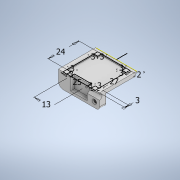
# Autodesk Inventor part: DisplayClipBase
Saved by Autodesk Inventor 2020.3 (Build 243373000, 373)
## iProperties
Created: 2020-07-13
Part Number: DisplayClipBase
Material: Generisch
Document SubType Name: Modeling
Designer: hpcwoess
Density: 1 g/cm^3
Appearance: Vorgabe
Author: hpcwoess
Autodesk Inventor part; units mm, degrees
ref_plane "YZ Plane" through (0, 0, 0) normal (1, 0, 0) x (0, 1, 0)
ref_plane "XZ Plane" through (0, 0, 0) normal (0, 1, 0) x (-1, 0, 0)
ref_plane "XY Plane" through (0, 0, 0) normal (0, 0, 1) x (1, 0, 0)
sketch "Skizze1" plane through (0, 0, 0) normal (0, 0, 1) x (1, 0, 0)
  line L0 (0, 0) -> (-11.6, 0)
  line L1 (-11.6, 0) -> (-11.6, 1.6)
  line L2 (-11.6, 1.6) -> (-9.6, 1.6)
  line L3 (-9.6, 1.6) -> (-9.6, 4.2)
  line L4 (-9.6, 4.2) -> (-16, 4.2)
  line L5 (-16, 4.2) -> (-16, 7)
  line L6 (-16, 7) -> (0, 7)
  line L7 (0, 7) -> (0, 0)
  dimension "d0" = 9.6
  dimension "d1" = 11.6
  dimension "d2" = 1.6
  dimension "d3" = 4.2
  dimension "d4" = 7
  dimension "d5" = 16
  constraints: 16 end point, 7 perpendicular, 1 horizontal
  measures "d0" distance between parallel lines of L7 L3
  measures "d1" distance of L0.start L0.end
  measures "d2" distance from line of L0.start L2
  measures "d3" distance between parallel lines of L4 L0
  measures "d4" distance between parallel lines of L0 L6
  measures "d5" distance between parallel lines of L7 L5
extrude "Extrusion1" add sketch "Skizze1" along normal blind 24
mirror "Spiegeln1" about plane through (0, 0, 0) normal (1, 0, 0) of "Extrusion1"
sketch "Skizze2" plane through (0, 0, 24) normal (0, 0, 1) x (1, 0, 0)
  line L0 (-16, 7) -> (-16, 4.2) projected
  line L1 (-16, 7) -> (16, 7)
  line L2 (16, 7) -> (16, -5)
  line L3 (16, -5) -> (-16, -5)
  line L4 (-16, -5) -> (-16, 7)
  line L5 (16, 7) -> (16, 4.2) projected
  point P0 (0, 0)
  dimension "d8" = 12
  constraints: 8 end point, 2 parallel, 1 collinear, 1 horizontal, 1 perpendicular
  measures "d8" distance between parallel lines of L3 L1
extrude "Extrusion2" add sketch "Skizze2" along normal blind 5
sketch "Skizze3" plane through (0, 0, 0) normal (1, 0, 0) x (0, 1, 0)
  line L0 (0, 0) -> (0, 24) projected
  line L1 (0.3, 3.5) -> (1.6, 3.5)
  line L2 (1.6, 3.5) -> (0, 11.5)
  line L3 (0, 11.5) -> (0, 4.0745)
  line L4 (1.6, 0) -> (0, 0) projected
  line L5 (0.3, 3.5) -> (0.3, 0)
  line L6 (0, 0) -> (0, 4.0745)
  line L7 (-5, 24) -> (4.2, 24) projected
  point P0 (0, 11.5)
  dimension "d12" = 8
  dimension "d13" = 1.7
  dimension "d14" = 0.3
  dimension "d20" = 20.5
  dimension "d65" = 1.3
  constraints: 10 end point, 2 perpendicular, 2 point on line, 1 horizontal, 1 vertical
  measures "d12" distance from line of L1 L2.end
  measures "d13" distance of L3.end L1.end
  measures "d14" distance between parallel lines of L0 L5
  measures "d20" distance between parallel lines of L1 L7
  measures "d65" distance of L1.start L1.end
extrude "Extrusion3" cut sketch "Skizze3" against normal mid plane 14
sketch "Skizze4" plane through (-16, 7, 0) normal (0, 1, 0) x (1, 0, 0)
  line L0 (3.5, -2) -> (28.5, -2)
  line L1 (28.5, -2) -> (28.5, -29)
  line L2 (28.5, -29) -> (3.5, -29)
  line L3 (3.5, -29) -> (3.5, -2)
  line L4 (16, 0) -> (16, 8.5337)
  line L5 (32, 0) -> (0, 0) projected
  line L6 (9.5, -26) -> (22.5, -26)
  line L7 (22.5, -26) -> (22.5, -29)
  line L8 (22.5, -29) -> (9.5, -29)
  line L9 (9.5, -29) -> (9.5, -26)
  line L10 (3.5, -29) -> (6.5, -29)
  line L11 (6.5, -29) -> (6.5, -26)
  line L12 (6.5, -26) -> (3.5, -26)
  line L13 (3.5, -26) -> (3.5, -29)
  line L14 (3.5, -2) -> (6.5, -2)
  line L15 (6.5, -2) -> (6.5, -5)
  line L16 (6.5, -5) -> (3.5, -5)
  line L17 (3.5, -5) -> (3.5, -2)
  line L18 (28.5, -29) -> (25.5, -29)
  line L19 (25.5, -29) -> (25.5, -26)
  line L20 (25.5, -26) -> (28.5, -26)
  line L21 (28.5, -26) -> (28.5, -29)
  line L22 (28.5, -2) -> (25.5, -2)
  line L23 (25.5, -2) -> (25.5, -5)
  line L24 (25.5, -5) -> (28.5, -5)
  line L25 (28.5, -5) -> (28.5, -2)
  point P0 (3.5, -26)
  dimension "d17" = 25
  dimension "d18" = 27
  dimension "d19" = 2
  dimension "d21" = 3
  dimension "d22" = 13
  dimension "d23" = 24
  dimension "d24" = 3
  dimension "d25" = 3
  dimension "d26" = 3
  dimension "d27" = 3
  dimension "d28" = 3
  dimension "d29" = 3
  dimension "d30" = 3
  dimension "d31" = 3
  constraints: 50 end point, 12 parallel, 6 horizontal, 6 perpendicular, 1 vertical, 2 other
  measures "d17" distance of L1.end L2.end
  measures "d18" distance of L0.end L1.end
  measures "d19" distance between parallel lines of L5 L0
  measures "d21" distance of L6.end L7.end
  measures "d22" distance of L7.end L8.end
  measures "d23" distance between parallel lines of L0 L6
  measures "d24" distance of L12.end L11.end
  measures "d25" distance of L11.end L10.end
  measures "d26" distance of L15.end L16.end
  measures "d27" distance of L14.end L15.end
  measures "d28" distance of L19.end L20.end
  measures "d29" distance of L18.end L19.end
  measures "d30" distance of L24.end L23.end
  measures "d31" distance of L23.end L22.end
extrude "Extrusion4" cut sketch "Skizze4" against normal blind 1 contours L0 L23 L24 L1 L20 L19 L2 L7 L6 L9 L11 L12 L3 L16 L15
extrude "Extrusion5" cut sketch "Skizze4" against normal blind 10 contours L9 L6 L7 L2
sketch "Skizze5" plane through (0, 0, 29) normal (0, 0, 1) x (1, 0, 0)
  circle A0 centre (12, -1) radius 1.75
  line L0 (-16, -5) -> (16, -5) projected
  line L1 (16, -5) -> (16, 7) projected
  point P0 (0, 0)
  dimension "d36" = 3.5
  dimension "d37" = 4
  dimension "d38" = 4
  constraints: 1 centre point
  measures "d36" diameter of A0
  measures "d37" distance from line of L0 A0.centre
  measures "d38" distance from line of A0.centre L1
extrude "Extrusion6" cut sketch "Skizze5" against normal blind 6.75
sketch "Skizze6" plane through (0, 0, 24) normal (0, 0, -1) x (-1, 0, 0)
  arc A0 (-11.6, 0.7037) -> (-10.5639, 0) centre (-12, -1) ccw projected
  line L0 (-10.2968, -3.95) -> (-13.7032, -3.95)
  line L1 (-13.7032, -3.95) -> (-15.4064, -1)
  line L2 (-15.4064, -1) -> (-13.7032, 1.95)
  line L3 (-13.7032, 1.95) -> (-10.2968, 1.95)
  line L4 (-10.2968, 1.95) -> (-8.5936, -1)
  line L5 (-8.5936, -1) -> (-10.2968, -3.95)
  point P0 (0, 0)
  dimension "d42" = 5.9
  constraints: 12 end point, 1 coincident, 1 horizontal, 13 other
  measures "d42" distance between parallel lines of L3 L0
extrude "Extrusion7" cut sketch "Skizze6" along normal mid plane 7.5
sketch "Skizze7" plane through (16, 4.2, 0) normal (1, 0, 0) x (0, 0, -1)
  line L0 (-29, 1.8) -> (-29, -7.2) projected
  circle A0 centre (-29, -0.2) radius 2
  line L1 (0, 2.8) -> (-29, 2.8) projected
  point P0 (0, -4.2)
  point P1 (-29, -2.2)
  dimension "d45" = 4
  dimension "d46" = 3
  constraints: 1 centre point, 1 point on line
  measures "d45" diameter of A0
  measures "d46" distance from line of A0.centre L1
extrude "Extrusion8" cut sketch "Skizze7" against normal blind 10 contours A0 L0 picked at (-28.3333, -0.2)
sketch "Skizze9" plane through (16, 4.2, 0) normal (1, 0, 0) x (0, 0, -1)
  line L0 (0, 0) -> (-24, 0) projected
  line L1 (0, 0) -> (-1, 0)
  line L2 (-1, 0) -> (-1, 1.6)
  line L3 (-1, 1.6) -> (0, 1.6)
  line L4 (0, 1.6) -> (0, 0)
  line L5 (0, 2.8) -> (-29, 2.8) projected
  line L6 (0, 2.8) -> (0, 0) projected
  line L7 (0, 2.8) -> (-0.2, 2.8)
  line L8 (-0.2, 2.8) -> (-0.2, 1.6)
  line L9 (-0.2, 1.6) -> (0, 1.6)
  line L10 (0, 1.6) -> (0, 2.8)
  point P0 (0, -4.2)
  dimension "d60" = 1
  dimension "d61" = 1.2
  dimension "d62" = 0.2
  constraints: 16 end point, 4 parallel, 2 horizontal, 2 perpendicular, 1 point on line
  measures "d60" distance of L2.end L3.end
  measures "d61" distance between parallel lines of L3 L5
  measures "d62" distance between parallel lines of L6 L8
extrude "Extrusion10" cut sketch "Skizze9" against normal up to surface (32 mm away)
fillet "Rundung1" radius 2.5 1 edges at (16, -5, 26.5)
fillet "Rundung2" radius 4 1 edges at (-16, -5, 26.5)
equation "\"d38\" = d37"
